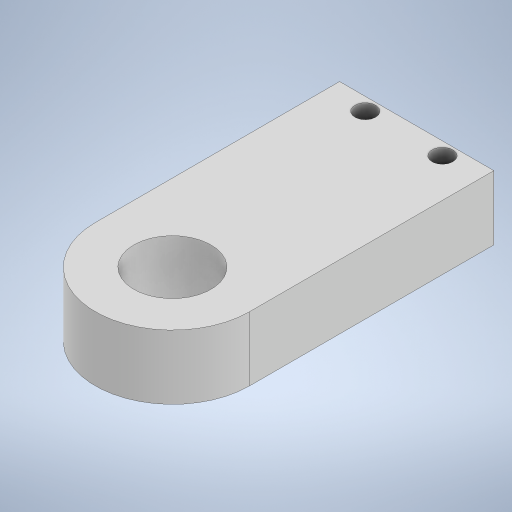
# Autodesk Inventor part: element2_obj4
Saved by Autodesk Inventor 2023.2 (Build 272271030, 271C)
## iProperties
Created: 2023-02-25
Part Number: element2_obj4
Material: Generic
Document SubType Name: Modeling
Designer: Cris Pat
Density: 1 g/cm^3
Appearance: Default
Author: Cris Pat
Autodesk Inventor part; units mm, degrees
ref_plane "YZ Plane" through (0, 0, 0) normal (1, 0, 0) x (0, 1, 0)
ref_plane "XZ Plane" through (0, 0, 0) normal (0, 1, 0) x (-1, 0, 0)
ref_plane "XY Plane" through (0, 0, 0) normal (0, 0, 1) x (1, 0, 0)
sketch "Sketch1" plane through (0, 0, 0) normal (0, 1, 0) x (-1, 0, 0)
  line L0 (30, -47.5) -> (-30, -47.5)
  line L1 (-30, -47.5) -> (-30, 47.5)
  arc A0 (30, 47.5) -> (-30, 47.5) centre (0, 47.5) ccw
  line L2 (30, 47.5) -> (30, -47.5)
  circle A1 centre (0, 47.5) radius 15
  point P0 (0, 0)
  point P1 (30, 0)
  dimension "d0" = 60
  dimension "d1" = 95
  dimension "d2" = 30
  constraints: 6 end point, 2 centre point, 2 horizontal alignment, 2 point on circle, 1 coincident, 1 horizontal, 1 midpoint, 1 parallel, 1 tangent, 1 vertical, 1 vertical alignment
  measures "d0" distance of L0.start L0.end
  measures "d1" distance of L0.end L1.end
  measures "d2" diameter of A1
extrude "Extrusion1" add sketch "Sketch1" along normal mid plane 25
sketch "Sketch2" plane through (0, 0, 0) normal (0, 1, 0) x (-1, 0, 0)
  line L0 (-30, -47.5) -> (-30, 47.5) construction
  arc A0 (30, 47.5) -> (-30, 47.5) centre (0, 47.5) ccw construction
  line L1 (30, 47.5) -> (30, -47.5) construction
  line L2 (30, -47.5) -> (-30, -47.5) construction
  circle A1 centre (0, 47.5) radius 15 construction
  line L3 (30, 47.5) -> (30, -47.5) construction
  line L4 (30, -37.5) -> (-30, -37.5) construction
  line L5 (-30, -47.5) -> (-30, 47.5) construction
  line L6 (0, -37.5) -> (0, -47.5) construction
  circle A2 centre (15, -42.5) radius 4.05
  circle A3 centre (-15, -42.5) radius 4.05
  point P0 (0, 0)
  point P1 (0, -42.5)
  dimension "d5" = 10
  dimension "d6" = 8.1
  dimension "d7" = 30
  constraints: 4 end point, 3 midpoint, 2 centre point, 2 point on line, 1 horizontal alignment, 1 perpendicular, 1 symmetric about line, 1 other
  measures "d5" distance between parallel lines of L2 L4
  measures "d6" diameter of A2
  measures "d7" distance of A3.centre A2.centre
extrude "Extrusion2" cut sketch "Sketch2" along normal through all both and the other way through all
body "Solid1"
